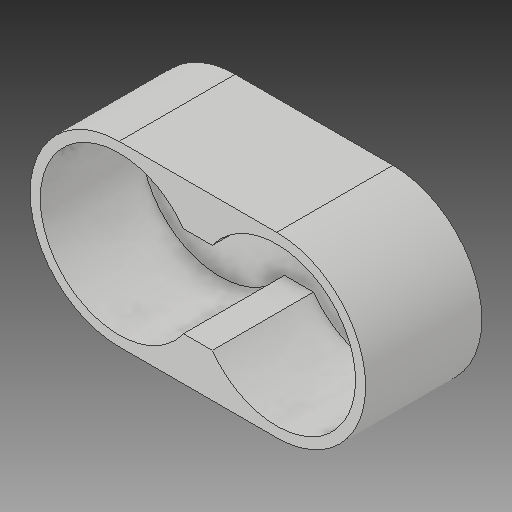
# Autodesk Inventor part: CaseBottom_CR123A
Saved by Autodesk Inventor 2018.1 (Build 221171000, 171)
## iProperties
Created: 2017-09-02
Part Number: CaseBottom_CR123A
Material: 一般
Document SubType Name: Modeling
Designer: sktom
Density: 1 g/cm^3
Appearance: 既定
Author: sktom
Autodesk Inventor part; units mm, degrees
ref_plane "YZ Plane" through (0, 0, 0) normal (1, 0, 0) x (0, 1, 0)
ref_plane "XZ Plane" through (0, 0, 0) normal (0, 1, 0) x (-1, 0, 0)
ref_plane "XY Plane" through (0, 0, 0) normal (0, 0, 1) x (1, 0, 0)
sketch "スケッチ1" plane through (0, 0, 0) normal (0, 0, 1) x (1, 0, 0)
  arc A0 (7.8, -7.8) -> (7.8, 7.8) centre (7.8, 0) ccw
  arc A1 (-7.8, 7.8) -> (-7.8, -7.8) centre (-7.8, 0) ccw
  line L0 (-7.8, 7.8) -> (7.8, 7.8)
  line L1 (7.8, -7.8) -> (-7.8, -7.8)
  line L2 (7.8, 8.8) -> (-7.8, 8.8)
  arc A2 (-7.8, 8.8) -> (-7.8, -8.8) centre (-7.8, 0) ccw
  line L3 (-7.8, -8.8) -> (7.8, -8.8)
  arc A3 (7.8, -8.8) -> (7.8, 8.8) centre (7.8, 0) ccw
  point P0 (0, 0)
  dimension "d0" = 15.6
  dimension "d1" = 15.6
  dimension "d2" = 7.8
  dimension "d3" = 1
  constraints: 8 end point, 8 point on circle, 4 centre point, 2 horizontal alignment, 2 parallel, 2 vertical alignment, 1 equal radius, 1 tangent, 3 other
  measures "d0" diameter of A0
  measures "d1" distance of L0.start L0.end
  measures "d2" horizontal distance of point (0, 0) L0.end
  measures "d3" distance between parallel lines of L0 L2
extrude "押し出し1" add sketch "スケッチ1" along normal blind 10
sketch "スケッチ2" plane through (0, 0, 0) normal (0, 0, -1) x (-1, 0, 0)
  line L0 (-7.8, 7.8) -> (7.8, 7.8) projected
  arc A0 (7.8, -7.8) -> (7.8, 7.8) centre (7.8, 0) ccw projected
  line L1 (7.8, -7.8) -> (-7.8, -7.8) projected
  arc A1 (-7.8, 7.8) -> (-7.8, -7.8) centre (-7.8, 0) ccw projected
  line L2 (-7.8, 8.8) -> (7.8, 8.8) projected
  arc A2 (-7.8, 8.8) -> (-7.8, -8.8) centre (-7.8, 0) ccw projected
  line L3 (7.8, -8.8) -> (-7.8, -8.8) projected
  arc A3 (7.8, -8.8) -> (7.8, 8.8) centre (7.8, 0) ccw projected
  point P0 (0, 0)
extrude "押し出し2" add sketch "スケッチ2" along normal blind 1.5 contours L0 A0 L1 A1 | L2 A3 L3 A2
sketch "スケッチ3" plane through (0, 0, 0) normal (0, 0, 1) x (1, 0, 0)
  arc A0 (-7.8, 7.8) -> (-7.8, -7.8) centre (-7.8, 0) ccw projected
  arc A1 (-7.8, -7.8) -> (-1.429, -4.5) centre (-7.8, 0) ccw
  arc A2 (7.8, -7.8) -> (7.8, 7.8) centre (7.8, 0) ccw projected
  arc A3 (1.429, -4.5) -> (7.8, -7.8) centre (7.8, 0) ccw
  line L0 (-1.429, -4.5) -> (1.429, -4.5)
  line L1 (7.8, -7.8) -> (-7.8, -7.8) projected
  line L2 (-7.8, -7.8) -> (7.8, -7.8)
  arc A4 (-1.429, 4.5) -> (-7.8, 7.8) centre (-7.8, 0) ccw
  arc A5 (7.8, 7.8) -> (1.429, 4.5) centre (7.8, 0) ccw
  line L3 (-1.429, 4.5) -> (1.429, 4.5)
  line L4 (-7.8, 7.8) -> (7.8, 7.8) projected
  line L5 (7.8, 7.8) -> (-7.8, 7.8)
  point P0 (0, 0)
  dimension "d9" = 9
  constraints: 9 point on circle, 8 end point, 4 centre point, 4 coincident, 3 tangent, 2 collinear, 2 parallel, 2 point on line, 1 horizontal
  measures "d9" distance between parallel lines of L3 L0
extrude "押し出し3" add sketch "スケッチ3" along normal up to surface (10 mm away) contours L4 A5 L3 A4 | A1 L0 A3 L1
